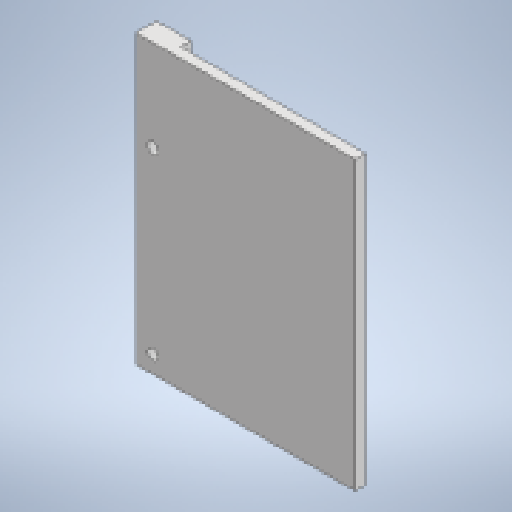
# Autodesk Inventor part: Lateral derecho
Saved by Autodesk Inventor 2024 (Build 280153000, 153)
## iProperties
Created: 2025-03-02
Part Number: Lateral derecho
Material: Genérico
Document SubType Name: Modeling
Designer: sergi
Density: 1 g/cm^3
Appearance: Valor por defecto
Author: sergi
Autodesk Inventor part; units mm, degrees
ref_plane "YZ Plane" through (0, 0, 0) normal (1, 0, 0) x (0, 1, 0)
ref_plane "Plano de trabajo7" through (63.9999, 14.8405, -83) normal (1, 0, 0) x (0, 1, 0)
sketch "Boceto2" plane through (0, 0, 0) normal (1, 0, 0) x (0, 1, 0)
  line L0 (0, 0) -> (-67, 0)
  line L1 (-67, 0) -> (-67, 3)
  line L2 (-67, 3) -> (0, 3)
  line L3 (0, 3) -> (0, 0)
  line L4 (16.65, -80) -> (16.65, 9) projected
  line L5 (0, 3) -> (16.65, 3)
  line L6 (16.65, 3) -> (16.65, 0)
  line L7 (16.65, 0) -> (0, 0)
  line L8 (0, 0) -> (0, 3)
  dimension "d2" = 67
  dimension "d3" = 3
  constraints: 16 end point, 4 parallel, 2 horizontal, 2 perpendicular, 1 point on line
  measures "d2" distance of L1.end L2.end
  measures "d3" distance of L0.end L1.end
extrude "Extrusión2" add sketch "Boceto2" along normal up to surface (63.9999 mm away)
sketch "Boceto8" plane through (0, -67, 3) normal (0, 0, 1) x (1, 0, 0)
  circle A0 centre (4.9999, 5) radius 2.1 projected
  circle A1 centre (4.9999, 57) radius 2.1 projected
  line L0 (-2.0001, 83.65) -> (-2.0001, 76.5) projected
  line L1 (-2.0001, 76.5) -> (-20.0001, 76.5) projected
  line L2 (-20.0001, 76.5) -> (-20.0001, 0) projected
  line L3 (9.9999, 0) -> (-20.0001, 0) projected
  line L4 (9.9999, 0) -> (9.9999, 83.65) projected
  line L5 (9.9999, 83.65) -> (-2.0001, 83.65) projected
  circle A2 centre (4.9999, 57) radius 1.6
  circle A3 centre (4.9999, 5) radius 1.6
  point P0 (0, 67)
  dimension "d31" = 3.2
  dimension "d32" = 3.2
  constraints: 2 centre point, 2 coincident
  measures "d31" diameter of A2
  measures "d32" diameter of A3
hole "Agujero3" at (4.9999, -10, 3) at (4.9999, -62, 3) direction (0, 0, -1) diameter 3.2 depth 5
sketch "Boceto9" plane through (0, -67, 0) normal (0, 0, -1) x (-1, 0, 0)
  line L0 (-9.9999, 83.65) -> (-9.9999, 0) projected
  line L1 (-63.9999, 0) -> (-9.9999, 0) projected
  circle A0 centre (-4.9999, 5) radius 1.6 projected
  circle A1 centre (-4.9999, 57) radius 1.6 projected
  line L2 (0, 0) -> (0, 83.65) projected
  line L3 (0, 83.65) -> (-63.9999, 83.65) projected
  line L4 (0, 0) -> (-63.9999, 0) projected
  line L5 (-63.9999, 83.65) -> (-63.9999, 0) projected
  line L6 (-9.9999, 83.65) -> (-32.9722, 83.65) projected
  line L7 (-40.0761, 83.65) -> (-63.9999, 83.65) projected
  line L8 (-32.9722, 83.65) -> (-29.7863, 64.5577) projected
  line L9 (-34.4654, 63.5184) -> (-40.0761, 83.65) projected
  arc A2 (-34.4654, 63.5184) -> (-29.7863, 64.5577) centre (-32.1535, 64.1627) ccw projected
  line L10 (-63.9999, 83.65) -> (-63.9999, 0) projected
  point P0 (0, 67)
  point P1 (-63.9999, 0)
  point P2 (-37.9999, 83.65)
extrude "Extrusión6" add sketch "Boceto9" along normal blind 3 contours L3 L2 L4 L0
sketch "Boceto10" plane through (65, -67, 0) normal (0, 0, -1) x (-1, 0, 0)
  line L0 (24.0001, 83.65) -> (24.0001, 86.65) projected
  line L1 (24.0001, 83.65) -> (27.0001, 83.65)
  line L2 (65, 83.65) -> (1.0001, 83.65) projected
  line L3 (35.8799, 60.5564) -> (35.8799, 64.1631) projected
  line L4 (35.8799, 60.4) -> (35.8799, 60.5564) projected
  line L5 (35.8799, 60.4) -> (33.8799, 60.4)
  line L6 (27.0001, 83.65) -> (30.0001, 83.65)
  line L7 (30.0001, 83.65) -> (33.8799, 60.4)
  line L8 (33.8799, 60.4) -> (33.4799, 60.4)
  line L9 (33.4799, 60.4) -> (27.0001, 83.65)
  point P0 (65, 67)
  point P1 (0, 83.65)
  dimension "d42" = 3
  dimension "d43" = 2
  dimension "d44" = 3
  dimension "d48" = 0.4
  constraints: 12 end point, 2 horizontal, 2 point on line
  measures "d42" distance of L0.start L1.end
  measures "d43" distance of L4.start L5.end
  measures "d44" distance of L1.end L6.end
  measures "d48" distance of L5.end L8.end
ref_plane "Plano de trabajo6" through (9.9999, -67, -72) normal (0, 0, 1) x (1, 0, 0)
extrude "Extrusión7" [suppressed]
fillet "Empalme1" [suppressed]
fillet "Empalme2" [suppressed]
